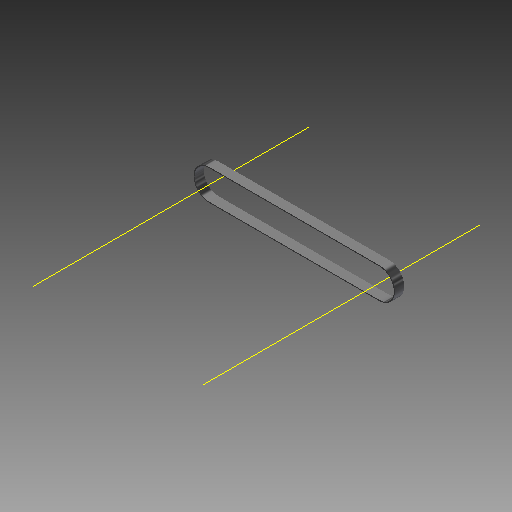
# Autodesk Inventor part: Synchronous Belt
Saved by Autodesk Inventor 2019.4 (Build 234330000, 330)
## iProperties
Created: 2020-02-08
Part Number: Synchronous Belt
Material: Rubber
Document SubType Name: Modeling
Designer: Paul Lefeuvre
Mass: 4.278 g
Surface Area: 101.2 cm^2
Volume: 4.6 cm^3
Density: 0.93 g/cm^3
Appearance: Rubber - Black - Version 1.1
CustomPartVersion: 1
Author: Paul Lefeuvre
Autodesk Inventor part; units mm, degrees
sketch "Sketch Path" plane through (0, 0, 0) normal (0, 0, 1) x (1, 0, 0)
  arc A0 (0, -48.2608) -> (0, -16.4298) centre (0, -32.3453) ccw
  arc A1 (-180, -16.4298) -> (-180, -48.2608) centre (-180, -32.3453) ccw
  line L0 (-180, -16.4298) -> (0, -16.4298)
  line L1 (0, -48.2608) -> (-180, -48.2608)
  constraints: 4 end point, 4 point on circle, 2 centre point
ref_plane "Cross Section Plane" through (0, -16.4298, 0) normal (-1, 0, 0) x (0, 0, 1)
ref_plane "Work Plane2" through (0, -32.3453, 0) normal (-1, 0, 0) x (0, 0, 1)
ref_plane "Work Plane3" through (-180, -32.3453, 0) normal (0.9511, -0.309, 0) x (0, 0, 1)
sketch "Cross Section" plane through (0, -16.4298, 0) normal (-1, 0, 0) x (0, 0, 1)
  line L0 (-5, 0.5) -> (5, 0.5)
  line L1 (5, 0.5) -> (5, -0.5)
  line L2 (5, -0.5) -> (-5, -0.5)
  line L3 (-5, -0.5) -> (-5, 0.5)
  line L4 (-5, 0) -> (5, 0) construction
  point P0 (0, 0)
  point P1 (0, 0)
  dimension "d0" = 10
  dimension "d4" = 0.5
  dimension "d5" = 0.5
  constraints: 10 end point, 3 midpoint, 2 parallel, 1 coincident, 1 horizontal, 1 perpendicular, 1 other
  measures "d0" distance between parallel lines of L1 L3
  measures "d4" distance between parallel lines of L2 L4
  measures "d5" distance between parallel lines of L4 L0
sweep "Belt" add profiles "Cross Section" path "Sketch Path"
equation "\"d0\" = da_B"
equation "\"d4\" = da_a"
equation "\"d5\" = da_a2"
equation "\"da_B\" = 10"
equation "\"da_pb\" = 5"
equation "\"da_a\" = 0.5"
equation "\"da_S\" = 2.65"
equation "\"da_Beta\" = 20deg"
equation "\"da_Ht\" = 1.2"
equation "\"da_H\" = 2.2"
equation "\"da_a2\" = 0.5"
body "Solid1"
